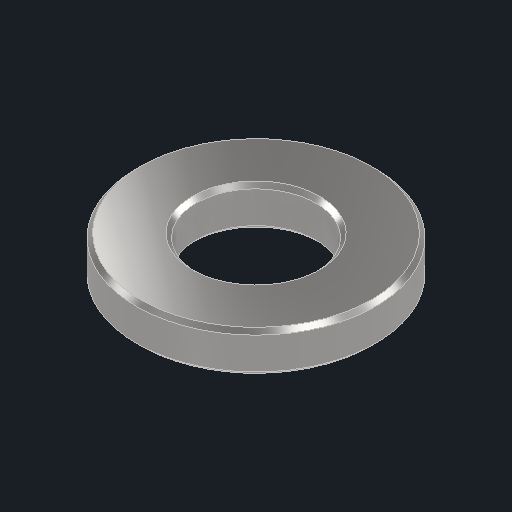
# Autodesk Inventor part: M6 Flat Washer - 12 OD x 2 Thick
Saved by Autodesk Inventor 2027.1 (Build 311270010, 270A)
## iProperties
Created: 2025-09-16
Part Number: M6 Flat Washer - 12 OD x 2 Thick
Material: Mild Steel S355 J2
Document SubType Name: Modeling
Designer: SD
Density: 7.85 g/cm^3
Appearance: Semi-Polished
Mass: 1.31396 g
Surface Area: 2.69493 cm^2
Volume: 0.167384 cm^3
Project: Automatic Tea Steeping mechanism
Description: Plain washers
BOM-Mass: 0.00131
BOM-Area: 0.000
Diameter: 12.000 mm
Thickness: 2.000 mm
Procurement: Buy
Preferred Material: Manufacturer Specification
Author: SD
Title: 6mm Washer
Autodesk Inventor part; units mm, degrees
ref_plane "YZ Plane" through (0, 0, 0) normal (1, 0, 0) x (0, 1, 0)
ref_plane "XZ Plane" through (0, 0, 0) normal (0, 1, 0) x (-1, 0, 0)
ref_plane "XY Plane" through (0, 0, 0) normal (0, 0, 1) x (1, 0, 0)
sketch "Sketch1" plane through (0, 0, 0) normal (0, 1, 0) x (-1, 0, 0)
  circle A0 centre (0, 0) radius 6
  circle A1 centre (0, 0) radius 3
  dimension "Diameter" = 12
  dimension "d1" = 6
  constraints: 2 centre point, 2 coincident
  measures "Diameter" diameter of A0
  measures "d1" diameter of A1
extrude "Extrusion1" add sketch "Sketch1" along normal blind 2
chamfer "Chamfer1" distance 0.2 angle 45 4 edges at (6, 2, 0) (3, 2, 0) (6, 0, 0) (3, 0, 0)
body "Solid1"
